Autodesk Fusion 360 part; units mm, degrees
(part 2 of 7)
  spline S300 degree 3 poles (-43.8986, 66.1485) (-43.8986, 66.1919) (-43.9124, 66.232) (-43.9361, 66.2647) knots 0 0 0 0 1 1 1 1
  spline S301 degree 3 poles (-43.9361, 66.2647) (-43.9588, 66.2897) (-43.9916, 66.3058) (-44.0281, 66.3058) knots 0 0 0 0 1 1 1 1
  line L172 (-44.0281, 66.3058) -> (-44.0291, 66.3058)
  spline S302 degree 3 poles (-44.0291, 66.3058) (-44.0304, 66.3058) (-44.0321, 66.3058) (-44.0335, 66.3058) knots 0 0 0 0 1 1 1 1
  spline S303 degree 3 poles (-44.0335, 66.3058) (-44.0697, 66.3058) (-44.1018, 66.2891) (-44.1235, 66.263) knots 0 0 0 0 1 1 1 1
  spline S304 degree 3 poles (-44.1235, 66.263) (-44.1441, 66.2339) (-44.1563, 66.1974) (-44.1563, 66.1582) knots 0 0 0 0 1 1 1 1
  spline S305 degree 3 poles (-44.1563, 66.1582) (-44.1563, 66.1516) (-44.1559, 66.1451) (-44.1553, 66.1389) knots 0 0 0 0 1 1 1 1
  line L173 (-44.1553, 66.1389) -> (-44.1573, 66.0745)
  spline S306 degree 3 poles (-44.1573, 66.0745) (-44.1654, 65.7573) (-44.1749, 65.398) (-44.5986, 65.398) knots 0 0 0 0 1 1 1 1
  spline S307 degree 3 poles (-44.5986, 65.398) (-44.8049, 65.398) (-45.0251, 65.5306) (-45.0251, 65.9016) knots 0 0 0 0 1 1 1 1
  line L174 (-45.0251, 65.9016) -> (-45.0251, 66.6018)
  line L175 (-45.0251, 66.6018) -> (-44.72, 66.6018)
  line L176 (-44.72, 66.6018) -> (-44.72, 65.9614)
  spline S308 degree 3 poles (-44.72, 65.9614) (-44.721, 65.9534) (-44.7214, 65.9444) (-44.7214, 65.935) knots 0 0 0 0 1 1 1 1
  spline S309 degree 3 poles (-44.7214, 65.935) (-44.7214, 65.8927) (-44.7109, 65.853) (-44.6923, 65.8184) knots 0 0 0 0 1 1 1 1
  line L177 (-44.6923, 65.8184) -> (-44.693, 65.8198)
  spline S310 degree 3 poles (-44.693, 65.8198) (-44.673, 65.7889) (-44.6389, 65.7685) (-44.6007, 65.7685) knots 0 0 0 0 1 1 1 1
  spline S311 degree 3 poles (-44.6007, 65.7685) (-44.5973, 65.7685) (-44.5942, 65.7685) (-44.5909, 65.7687) knots 0 0 0 0 1 1 1 1
  line L178 (-44.5909, 65.7687) -> (-44.5875, 65.7687)
  spline S312 degree 3 poles (-44.5875, 65.7687) (-44.5395, 65.7687) (-44.4989, 65.8006) (-44.4847, 65.8451) knots 0 0 0 0 1 1 1 1
  spline S313 degree 3 poles (-44.4847, 65.8451) (-44.4738, 65.8802) (-44.4674, 65.9197) (-44.4674, 65.9606) knots 0 0 0 0 1 1 1 1
  spline S314 degree 3 poles (-44.4674, 65.9606) (-44.4674, 65.9677) (-44.4677, 65.9748) (-44.4681, 65.9818) knots 0 0 0 0 1 1 1 1
  line L179 (-44.4681, 65.9818) -> (-44.4681, 65.9807)
  line L180 (-44.4681, 65.9807) -> (-44.4633, 66.1712)
  spline S315 degree 3 poles (-44.4633, 66.1712) (-44.465, 66.1872) (-44.4661, 66.206) (-44.4661, 66.2247) knots 0 0 0 0 1 1 1 1
  spline S316 degree 3 poles (-44.4661, 66.2247) (-44.4661, 66.3556) (-44.4218, 66.476) (-44.3474, 66.5708) knots 0 0 0 0 1 1 1 1
  line L181 (-44.3474, 66.5708) -> (-44.348, 66.5696)
  spline S317 degree 3 poles (-44.348, 66.5696) (-44.3399, 66.5801) (-44.3311, 66.5891) (-44.3213, 66.5971) knots 0 0 0 0 1 1 1 1
  line L182 (-44.3213, 66.5971) -> (-43.7758, 66.6017)
  spline S318 degree 3 poles (-43.7758, 66.6017) (-43.6615, 66.5006) (-43.5895, 66.3517) (-43.5895, 66.1855) knots 0 0 0 0 1 1 1 1
  spline S319 degree 3 poles (-43.5895, 66.1855) (-43.5895, 66.164) (-43.5908, 66.1428) (-43.5929, 66.1223) knots 0 0 0 0 1 1 1 1
  line L183 (-43.5929, 66.1223) -> (-43.5925, 66.1249)
  line L184 (-43.5925, 64.7542) -> (-43.5925, 64.0697)
  line L185 (-43.5925, 64.0697) -> (-43.9003, 64.0697)
  line L186 (-43.9003, 64.0697) -> (-43.9003, 64.7506)
  spline S320 degree 3 poles (-43.9003, 64.7506) (-43.8993, 64.7583) (-43.8986, 64.7673) (-43.8986, 64.7764) knots 0 0 0 0 1 1 1 1
  spline S321 degree 3 poles (-43.8986, 64.7764) (-43.8986, 64.8205) (-43.9124, 64.8614) (-43.9361, 64.8948) knots 0 0 0 0 1 1 1 1
  spline S322 degree 3 poles (-43.9361, 64.8948) (-43.9588, 64.9194) (-43.9919, 64.935) (-44.0281, 64.935) knots 0 0 0 0 1 1 1 1
  line L187 (-44.0281, 64.935) -> (-44.0291, 64.935)
  spline S323 degree 3 poles (-44.0291, 64.935) (-44.0298, 64.935) (-44.0308, 64.935) (-44.0315, 64.935) knots 0 0 0 0 1 1 1 1
  spline S324 degree 3 poles (-44.0315, 64.935) (-44.068, 64.935) (-44.1012, 64.9183) (-44.1235, 64.8922) knots 0 0 0 0 1 1 1 1
  spline S325 degree 3 poles (-44.1235, 64.8922) (-44.1441, 64.8627) (-44.1563, 64.8257) (-44.1563, 64.7857) knots 0 0 0 0 1 1 1 1
  spline S326 degree 3 poles (-44.1563, 64.7857) (-44.1563, 64.7791) (-44.1559, 64.7725) (-44.1553, 64.7662) knots 0 0 0 0 1 1 1 1
  line L188 (-44.1553, 64.7662) -> (-44.1573, 64.7024)
  spline S327 degree 3 poles (-44.1573, 64.7024) (-44.1654, 64.3862) (-44.1749, 64.0274) (-44.5986, 64.0274) knots 0 0 0 0 1 1 1 1
  spline S328 degree 3 poles (-44.5986, 64.0274) (-44.8049, 64.0274) (-45.0251, 64.1593) (-45.0251, 64.5296) knots 0 0 0 0 1 1 1 1
  line L189 (-45.0251, 64.5296) -> (-45.0251, 65.2335)
  line L190 (-45.0251, 65.2335) -> (-44.72, 65.2335)
  line L191 (-44.72, 65.2335) -> (-44.72, 64.5894)
  spline S329 degree 3 poles (-44.72, 64.5894) (-44.7211, 64.5814) (-44.7214, 64.5724) (-44.7214, 64.5633) knots 0 0 0 0 1 1 1 1
  spline S330 degree 3 poles (-44.7214, 64.5633) (-44.7214, 64.5213) (-44.7109, 64.4818) (-44.6923, 64.4474) knots 0 0 0 0 1 1 1 1
  line L192 (-44.6923, 64.4474) -> (-44.693, 64.4489)
  spline S331 degree 3 poles (-44.693, 64.4489) (-44.671, 64.4165) (-44.6352, 64.3956) (-44.5946, 64.3956) knots 0 0 0 0 1 1 1 1
  spline S332 degree 3 poles (-44.5946, 64.3956) (-44.5445, 64.3956) (-44.5016, 64.4273) (-44.4837, 64.4717) knots 0 0 0 0 1 1 1 1
  spline S333 degree 3 poles (-44.4837, 64.4717) (-44.4728, 64.5072) (-44.4664, 64.5467) (-44.4664, 64.5881) knots 0 0 0 0 1 1 1 1
  spline S334 degree 3 poles (-44.4664, 64.5881) (-44.4664, 64.5954) (-44.4667, 64.6029) (-44.4671, 64.6103) knots 0 0 0 0 1 1 1 1
  line L193 (-44.4671, 64.6103) -> (-44.4671, 64.6091)
  line L194 (-44.4671, 64.6091) -> (-44.4624, 64.7984)
  spline S335 degree 3 poles (-44.4624, 64.7984) (-44.4641, 64.8143) (-44.4647, 64.8327) (-44.4647, 64.8511) knots 0 0 0 0 1 1 1 1
  spline S336 degree 3 poles (-44.4647, 64.8511) (-44.4647, 64.9829) (-44.4204, 65.1044) (-44.346, 65.2003) knots 0 0 0 0 1 1 1 1
  line L195 (-44.346, 65.2003) -> (-44.347, 65.1991)
  spline S337 degree 3 poles (-44.347, 65.1991) (-44.276, 65.2652) (-44.1817, 65.3058) (-44.0778, 65.3058) knots 0 0 0 0 1 1 1 1
  spline S338 degree 3 poles (-44.0778, 65.3058) (-44.066, 65.3058) (-44.0538, 65.3049) (-44.0423, 65.304) knots 0 0 0 0 1 1 1 1
  line L196 (-44.0423, 65.304) -> (-44.044, 65.304)
  spline S339 degree 3 poles (-44.044, 65.304) (-43.7454, 65.3049) (-43.5932, 65.1193) (-43.5932, 64.7531) knots 0 0 0 0 1 1 1 1
  line L197 (-43.5932, 64.7531) -> (-43.5925, 64.7542)
  line L198 (-43.5925, 63.8593) -> (-43.5925, 62.6862)
  line L199 (-43.5925, 62.6862) -> (-45.0254, 62.6862)
  line L200 (-45.0254, 62.6862) -> (-45.0254, 63.8582)
  line L201 (-45.0254, 63.8582) -> (-44.7295, 63.8582)
  line L202 (-44.7295, 63.8582) -> (-44.7295, 63.0367)
  line L203 (-44.7295, 63.0367) -> (-44.4691, 63.0367)
  line L204 (-44.4691, 63.0367) -> (-44.4691, 63.8392)
  line L205 (-44.4691, 63.8392) -> (-44.1773, 63.8392)
  line L206 (-44.1773, 63.8392) -> (-44.1773, 63.0367)
  line L207 (-44.1773, 63.0367) -> (-43.8925, 63.0367)
  line L208 (-43.8925, 63.0367) -> (-43.8911, 63.8593)
  line L209 (-43.8911, 63.8593) -> (-43.5935, 63.8593)
  line L210 (-43.5935, 63.8593) -> (-43.5925, 63.8593)
  line L211 (-46.0566, 64.5431) -> (-46.0566, 63.8278)
  line L212 (-46.0566, 63.8278) -> (-46.3758, 63.691)
  line L213 (-46.3758, 63.691) -> (-46.3758, 62.9615)
  line L214 (-46.3758, 62.9615) -> (-46.0566, 62.8289)
  line L215 (-46.0566, 62.8289) -> (-46.0566, 62.4179)
  spline S340 degree 3 poles (-46.0566, 62.4179) (-46.0559, 62.4064) (-46.0556, 62.3929) (-46.0556, 62.3793) knots 0 0 0 0 1 1 1 1
  spline S341 degree 3 poles (-46.0556, 62.3793) (-46.0556, 62.2009) (-46.1154, 62.0368) (-46.2159, 61.907) knots 0 0 0 0 1 1 1 1
  line L216 (-46.2159, 61.907) -> (-46.2148, 61.9087)
  spline S342 degree 3 poles (-46.2148, 61.9087) (-46.3423, 61.7903) (-46.5118, 61.7181) (-46.6981, 61.7181) knots 0 0 0 0 1 1 1 1
  spline S343 degree 3 poles (-46.6981, 61.7181) (-46.7204, 61.7181) (-46.7428, 61.7192) (-46.7644, 61.7212) knots 0 0 0 0 1 1 1 1
  line L217 (-46.7644, 61.7212) -> (-46.7617, 61.721)
  spline S344 degree 3 poles (-46.7617, 61.721) (-46.7806, 61.7192) (-46.8026, 61.7181) (-46.8249, 61.7181) knots 0 0 0 0 1 1 1 1
  spline S345 degree 3 poles (-46.8249, 61.7181) (-47.0157, 61.7181) (-47.1895, 61.791) (-47.3221, 61.9111) knots 0 0 0 0 1 1 1 1
  spline S346 degree 3 poles (-47.3221, 61.9111) (-47.4269, 62.0343) (-47.4912, 62.1975) (-47.4912, 62.3763) knots 0 0 0 0 1 1 1 1
  spline S347 degree 3 poles (-47.4912, 62.3763) (-47.4912, 62.4002) (-47.4902, 62.4234) (-47.4878, 62.4467) knots 0 0 0 0 1 1 1 1
  line L218 (-47.4878, 62.4467) -> (-47.4881, 62.4438)
  line L219 (-47.4881, 62.4438) -> (-47.4881, 62.784)
  line L220 (-47.4881, 62.784) -> (-47.1827, 62.784)
  line L221 (-47.1827, 62.784) -> (-47.1827, 62.4508)
  spline S348 degree 3 poles (-47.1827, 62.4508) (-47.1844, 62.4384) (-47.1854, 62.4236) (-47.1854, 62.4088) knots 0 0 0 0 1 1 1 1
  spline S349 degree 3 poles (-47.1854, 62.4088) (-47.1854, 62.3203) (-47.1523, 62.2402) (-47.0979, 62.1801) knots 0 0 0 0 1 1 1 1
  spline S350 degree 3 poles (-47.0979, 62.1801) (-47.0187, 62.1165) (-46.9173, 62.0781) (-46.8074, 62.0781) knots 0 0 0 0 1 1 1 1
  spline S351 degree 3 poles (-46.8074, 62.0781) (-46.7955, 62.0781) (-46.7837, 62.0783) (-46.7722, 62.0792) knots 0 0 0 0 1 1 1 1
  line L222 (-46.7722, 62.0792) -> (-46.7739, 62.0792)
  spline S352 degree 3 poles (-46.7739, 62.0792) (-46.761, 62.0781) (-46.7458, 62.0772) (-46.7306, 62.0772) knots 0 0 0 0 1 1 1 1
  spline S353 degree 3 poles (-46.7306, 62.0772) (-46.6203, 62.0772) (-46.5185, 62.1144) (-46.4364, 62.1768) knots 0 0 0 0 1 1 1 1
  line L223 (-46.4364, 62.1768) -> (-46.4377, 62.1757)
  spline S354 degree 3 poles (-46.4377, 62.1757) (-46.391, 62.2344) (-46.3626, 62.3096) (-46.3626, 62.3922) knots 0 0 0 0 1 1 1 1
  spline S355 degree 3 poles (-46.3626, 62.3922) (-46.3626, 62.4023) (-46.363, 62.4121) (-46.364, 62.4217) knots 0 0 0 0 1 1 1 1
  line L224 (-46.364, 62.4217) -> (-46.364, 62.4203)
  line L225 (-46.364, 62.4203) -> (-46.364, 62.578)
  line L226 (-46.364, 62.578) -> (-47.4902, 63.0747)
  line L227 (-47.4902, 63.0747) -> (-47.4902, 63.6022)
  line L228 (-47.4902, 63.6022) -> (-46.1374, 64.1968)
  line L229 (-46.1374, 64.1968) -> (-47.4902, 64.1968)
  line L230 (-47.4902, 64.1968) -> (-47.4902, 64.7316)
  line L231 (-47.4902, 64.7316) -> (-46.4932, 65.3489)
  line L232 (-46.4932, 65.3489) -> (-47.4902, 65.3489)
  line L233 (-47.4902, 65.3489) -> (-47.4902, 65.7097)
  line L234 (-47.4902, 65.7097) -> (-46.059, 65.7097)
  line L235 (-46.059, 65.7097) -> (-46.059, 65.2088)
  line L236 (-46.059, 65.2088) -> (-47.1337, 64.5423)
  line L237 (-47.1337, 64.5423) -> (-46.059, 64.5423)
  line L238 (-46.059, 64.5423) -> (-46.0566, 64.5431)
  line L239 (-47.2463, 63.3286) -> (-46.6755, 63.0867)
  line L240 (-46.6755, 63.0867) -> (-46.6755, 63.5715)
  line L241 (-46.6755, 63.5715) -> (-47.2463, 63.3286)
  line L242 (-46.0573, 59.9275) -> (-46.0573, 59.5762)
  line L243 (-46.0573, 59.5762) -> (-47.4892, 59.5762)
  line L244 (-47.4892, 59.5762) -> (-47.4892, 60.3842)
  spline S356 degree 3 poles (-47.4892, 60.3842) (-47.4919, 60.4092) (-47.4932, 60.4384) (-47.4932, 60.4679) knots 0 0 0 0 1 1 1 1
  spline S357 degree 3 poles (-47.4932, 60.4679) (-47.4932, 60.5917) (-47.4665, 60.7095) (-47.4185, 60.815) knots 0 0 0 0 1 1 1 1
  line L245 (-47.4185, 60.815) -> (-47.4205, 60.8097)
  spline S358 degree 3 poles (-47.4205, 60.8097) (-47.362, 60.917) (-47.2521, 60.9882) (-47.1259, 60.9882) knots 0 0 0 0 1 1 1 1
  spline S359 degree 3 poles (-47.1259, 60.9882) (-47.1178, 60.9882) (-47.11, 60.9879) (-47.1023, 60.9873) knots 0 0 0 0 1 1 1 1
  line L246 (-47.1023, 60.9873) -> (-47.1033, 60.9873)
  line L247 (-47.1033, 60.9873) -> (-47.0928, 60.9873)
  spline S360 degree 3 poles (-47.0928, 60.9873) (-46.9281, 60.9873) (-46.7864, 60.8867) (-46.7228, 60.7423) knots 0 0 0 0 1 1 1 1
  line L248 (-46.7228, 60.7423) -> (-46.7218, 60.7394)
  spline S361 degree 3 poles (-46.7218, 60.7394) (-46.6961, 60.8092) (-46.6548, 60.8679) (-46.6021, 60.9126) knots 0 0 0 0 1 1 1 1
  line L249 (-46.6021, 60.9126) -> (-46.6014, 60.9134)
  spline S362 degree 3 poles (-46.6014, 60.9134) (-46.5405, 60.9515) (-46.4668, 60.9745) (-46.3877, 60.9745) knots 0 0 0 0 1 1 1 1
  spline S363 degree 3 poles (-46.3877, 60.9745) (-46.3704, 60.9745) (-46.3535, 60.9733) (-46.3366, 60.9713) knots 0 0 0 0 1 1 1 1
  line L250 (-46.3366, 60.9713) -> (-46.3386, 60.9716)
  line L251 (-46.3386, 60.9716) -> (-46.0576, 60.9716)
  line L252 (-46.0576, 60.9716) -> (-46.0576, 60.6173)
  line L253 (-46.0576, 60.6173) -> (-46.2382, 60.6158)
  line L254 (-46.2382, 60.6158) -> (-46.2652, 60.6158)
  spline S364 degree 3 poles (-46.2652, 60.6158) (-46.2805, 60.6179) (-46.298, 60.6194) (-46.3163, 60.6194) knots 0 0 0 0 1 1 1 1
  spline S365 degree 3 poles (-46.3163, 60.6194) (-46.3907, 60.6194) (-46.46, 60.5975) (-46.5185, 60.5594) knots 0 0 0 0 1 1 1 1
  line L255 (-46.5185, 60.5594) -> (-46.5169, 60.5603)
  spline S366 degree 3 poles (-46.5169, 60.5603) (-46.5574, 60.5037) (-46.5821, 60.4325) (-46.5821, 60.3555) knots 0 0 0 0 1 1 1 1
  spline S367 degree 3 poles (-46.5821, 60.3555) (-46.5821, 60.3374) (-46.5808, 60.3195) (-46.5781, 60.302) knots 0 0 0 0 1 1 1 1
  line L256 (-46.5781, 60.302) -> (-46.5784, 60.3043)
  line L257 (-46.5784, 60.3043) -> (-46.5784, 59.9277)
  line L258 (-46.5784, 59.9277) -> (-46.0573, 59.9275)
  line L259 (-47.1912, 59.9275) -> (-46.8733, 59.9275)
  line L260 (-46.8733, 59.9275) -> (-46.8733, 60.3536)
  spline S368 degree 3 poles (-46.8733, 60.3536) (-46.8723, 60.3638) (-46.8716, 60.3757) (-46.8716, 60.3873) knots 0 0 0 0 1 1 1 1
  spline S369 degree 3 poles (-46.8716, 60.3873) (-46.8716, 60.4384) (-46.8831, 60.4863) (-46.9038, 60.529) knots 0 0 0 0 1 1 1 1
  line L261 (-46.9038, 60.529) -> (-46.9031, 60.5272)
  spline S370 degree 3 poles (-46.9031, 60.5272) (-46.9295, 60.5713) (-46.9761, 60.6002) (-47.0292, 60.6002) knots 0 0 0 0 1 1 1 1
  spline S371 degree 3 poles (-47.0292, 60.6002) (-47.0323, 60.6002) (-47.0356, 60.6002) (-47.0387, 60.5996) knots 0 0 0 0 1 1 1 1
  spline S372 degree 3 poles (-47.0387, 60.5996) (-47.0414, 60.6002) (-47.0441, 60.6002) (-47.0472, 60.6002) knots 0 0 0 0 1 1 1 1
  spline S373 degree 3 poles (-47.0472, 60.6002) (-47.0982, 60.6002) (-47.1425, 60.5703) (-47.1645, 60.5265) knots 0 0 0 0 1 1 1 1
  spline S374 degree 3 poles (-47.1645, 60.5265) (-47.1824, 60.4842) (-47.1929, 60.4359) (-47.1929, 60.385) knots 0 0 0 0 1 1 1 1
  spline S375 degree 3 poles (-47.1929, 60.385) (-47.1929, 60.3759) (-47.1926, 60.3669) (-47.1919, 60.3582) knots 0 0 0 0 1 1 1 1
  line L262 (-47.1919, 60.3582) -> (-47.1919, 60.3593)
  line L263 (-47.1919, 60.3593) -> (-47.1912, 59.9275)
  line L264 (-46.0573, 56.208) -> (-46.0573, 55.4944)
  line L265 (-46.0573, 55.4944) -> (-46.3765, 55.3593)
  line L266 (-46.3765, 55.3593) -> (-46.3765, 54.6276)
  line L267 (-46.3765, 54.6276) -> (-46.0573, 54.4916)
  line L268 (-46.0573, 54.4916) -> (-46.0573, 54.1098)
  line L269 (-46.0573, 54.1098) -> (-47.4892, 54.7391)
  line L270 (-47.4892, 54.7391) -> (-47.4892, 55.2608)
  line L271 (-47.4892, 55.2608) -> (-46.134, 55.8581)
  line L272 (-46.134, 55.8581) -> (-47.4892, 55.8581)
  line L273 (-47.4892, 55.8581) -> (-47.4892, 56.4312)
  line L274 (-47.4892, 56.4312) -> (-46.5182, 56.8907)
  line L275 (-46.5182, 56.8907) -> (-47.4892, 57.3131)
  line L276 (-47.4892, 57.3131) -> (-47.4892, 57.898)
  line L277 (-47.4892, 57.898) -> (-46.0579, 57.898)
  line L278 (-46.0579, 57.898) -> (-46.0579, 57.537)
  line L279 (-46.0579, 57.537) -> (-47.178, 57.5364)
  line L280 (-47.178, 57.5364) -> (-46.0576, 57.0272)
  line L281 (-46.0576, 57.0272) -> (-46.0576, 56.719)
  line L282 (-46.0576, 56.719) -> (-47.1797, 56.2084)
  line L283 (-47.1797, 56.2084) -> (-46.0573, 56.208)
  line L284 (-47.2463, 54.9918) -> (-46.6755, 54.7526)
  line L285 (-46.6755, 54.7526) -> (-46.6755, 55.2322)
  line L286 (-46.6755, 55.2322) -> (-47.2463, 54.9918)
  line L287 (-46.0576, 61.5477) -> (-46.0576, 61.1895)
  line L288 (-46.0576, 61.1895) -> (-47.4892, 61.1895)
  line L289 (-47.4892, 61.1895) -> (-47.4892, 61.548)
  line L290 (-47.4892, 61.548) -> (-46.0576, 61.5477)
  line L291 (-46.0576, 59.3312) -> (-46.0576, 58.16)
  line L292 (-46.0576, 58.16) -> (-47.4892, 58.16)
  line L293 (-47.4892, 58.16) -> (-47.4892, 59.3332)
  line L294 (-47.4892, 59.3332) -> (-47.1916, 59.3332)
  line L295 (-47.1916, 59.3332) -> (-47.1916, 58.5114)
  line L296 (-47.1916, 58.5114) -> (-46.9335, 58.5114)
  line L297 (-46.9335, 58.5114) -> (-46.9335, 59.3135)
  line L298 (-46.9335, 59.3135) -> (-46.6396, 59.3135)
  line L299 (-46.6396, 59.3135) -> (-46.6396, 58.5106)
  line L300 (-46.6396, 58.5106) -> (-46.3535, 58.5106)
  line L301 (-46.3535, 58.5106) -> (-46.3535, 59.3326)
  line L302 (-46.3535, 59.3326) -> (-46.0579, 59.3326)
  line L303 (-46.0579, 59.3326) -> (-46.0576, 59.3312)
  ellipse E0 centre (-45.5414, 48.1762) end of major axis (-45.5414, 50.128) minor radius 1.9518
  spline S376 degree 3 poles (-45.5413, 52.5482) (-44.4633, 52.5482) (-43.5894, 51.6744) (-43.5894, 50.5965) knots 0 0 0 0 1 1 1 1
  spline S377 degree 3 poles (-43.5894, 50.5965) (-43.5894, 49.5184) (-44.4633, 48.6446) (-45.5413, 48.6446) knots 0 0 0 0 1 1 1 1
  spline S378 degree 3 poles (-45.5413, 48.6446) (-46.6193, 48.6446) (-47.4931, 49.5184) (-47.4931, 50.5965) knots 0 0 0 0 1 1 1 1
  spline S379 degree 3 poles (-47.4931, 50.5965) (-47.4931, 51.6744) (-46.6193, 52.5482) (-45.5413, 52.5482) knots 0 0 0 0 1 1 1 1
  spline S380 degree 3 poles (-47.0729, 49.3863) (-46.7154, 48.9344) (-46.1622, 48.6446) (-45.5413, 48.6446) knots 0 0 0 0 1 1 1 1
  spline S381 degree 3 poles (-45.5413, 48.6446) (-44.9205, 48.6446) (-44.3673, 48.9344) (-44.0098, 49.3863) knots 0 0 0 0 1 1 1 1
  spline S382 degree 3 poles (-44.0098, 49.3863) (-44.3673, 49.8381) (-44.9205, 50.128) (-45.5414, 50.128) knots 0 0 0 0 1 1 1 1
  spline S383 degree 3 poles (-45.5414, 50.128) (-46.1622, 50.128) (-46.7154, 49.8381) (-47.0729, 49.3863) knots 0 0 0 0 1 1 1 1
  spline S384 degree 3 poles (-46.3077, 38.5284) (-46.3077, 38.1545) (-46.5644, 37.8257) (-47.006, 37.8257) knots 0 0 0 0 1 1 1 1
  spline S385 degree 3 poles (-47.006, 37.8257) (-47.4464, 37.8257) (-47.7032, 38.1555) (-47.7032, 38.5284) knots 0 0 0 0 1 1 1 1
  spline S386 degree 3 poles (-47.7032, 38.5284) (-47.7032, 38.8981) (-47.4454, 39.227) (-47.006, 39.227) knots 0 0 0 0 1 1 1 1
  spline S387 degree 3 poles (-47.006, 39.227) (-46.5644, 39.2279) (-46.3077, 38.8981) (-46.3077, 38.5284) knots 0 0 0 0 1 1 1 1
  spline S388 degree 3 poles (-47.5409, 38.5285) (-47.5409, 38.249) (-47.3272, 38.0266) (-47.0059, 38.0266) knots 0 0 0 0 1 1 1 1
  spline S389 degree 3 poles (-47.0059, 38.0266) (-46.6847, 38.0266) (-46.4688, 38.249) (-46.4688, 38.5285) knots 0 0 0 0 1 1 1 1
  spline S390 degree 3 poles (-46.4688, 38.5285) (-46.4688, 38.7971) (-46.6847, 39.026) (-47.0059, 39.026) knots 0 0 0 0 1 1 1 1
  spline S391 degree 3 poles (-47.0059, 39.026) (-47.3272, 39.026) (-47.5409, 38.7971) (-47.5409, 38.5285) knots 0 0 0 0 1 1 1 1
  spline S392 degree 3 poles (-45.0228, 38.5327) (-46.1175, 37.4503) (-47.0023, 36.1744) (-47.6323, 34.7695) knots 0 0 0 0 1 1 1 1
  spline S393 degree 3 poles (-47.6323, 34.7695) (-48.2605, 33.3622) (-48.5856, 31.8384) (-48.5863, 30.2971) knots 0 0 0 0 1 1 1 1
  spline S394 degree 3 poles (-48.5863, 30.2971) (-48.5854, 28.5466) (-48.1674, 26.8215) (-47.3669, 25.2648) knots 0 0 0 0 1 1 1 1
  spline S395 degree 3 poles (-47.3669, 25.2648) (-46.5902, 23.7378) (-45.4837, 22.3687) (-44.0753, 21.1974) knots 0 0 0 0 1 1 1 1
  spline S396 degree 3 poles (-44.0753, 21.1974) (-41.2068, 18.8097) (-37.4027, 17.4944) (-33.3623, 17.4944) knots 0 0 0 0 1 1 1 1
  spline S397 degree 3 poles (-33.3623, 17.4944) (-28.8523, 17.4944) (-24.6024, 19.1589) (-21.7018, 22.0614) knots 0 0 0 0 1 1 1 1
  spline S398 degree 3 poles (-21.7018, 22.0614) (-20.6065, 23.1441) (-19.7215, 24.4204) (-19.0911, 25.8257) knots 0 0 0 0 1 1 1 1
  spline S399 degree 3 poles (-19.0911, 25.8257) (-18.4623, 27.2329) (-18.1373, 28.7569) (-18.1373, 30.2982) knots 0 0 0 0 1 1 1 1
  spline S400 degree 3 poles (-18.1373, 30.2982) (-18.1373, 31.8395) (-18.4623, 33.3636) (-19.0911, 34.7706) knots 0 0 0 0 1 1 1 1
  spline S401 degree 3 poles (-19.0911, 34.7706) (-19.6971, 36.1429) (-20.5769, 37.4088) (-21.7018, 38.5338) knots 0 0 0 0 1 1 1 1
  spline S402 degree 3 poles (-21.7018, 38.5338) (-24.6024, 41.4363) (-28.8523, 43.1009) (-33.3623, 43.1009) knots 0 0 0 0 1 1 1 1
  spline S403 degree 3 poles (-33.3623, 43.1009) (-37.8711, 43.0998) (-42.1211, 41.4352) (-45.0228, 38.5327) knots 0 0 0 0 1 1 1 1
  spline S404 degree 3 poles (-18.4058, 30.2971) (-18.4064, 31.8009) (-18.7229, 33.2877) (-19.335, 34.661) knots 0 0 0 0 1 1 1 1
  spline S405 degree 3 poles (-19.335, 34.661) (-19.952, 36.0356) (-20.8183, 37.2838) (-21.8898, 38.3427) knots 0 0 0 0 1 1 1 1
  spline S406 degree 3 poles (-21.8898, 38.3427) (-24.741, 41.1946) (-28.9232, 42.8323) (-33.3623, 42.8323) knots 0 0 0 0 1 1 1 1
  spline S407 degree 3 poles (-33.3623, 42.8323) (-37.8002, 42.8323) (-41.9804, 41.1957) (-44.8327, 38.3427) knots 0 0 0 0 1 1 1 1
  spline S408 degree 3 poles (-44.8327, 38.3427) (-45.9051, 37.2846) (-46.7714, 36.0361) (-47.3874, 34.661) knots 0 0 0 0 1 1 1 1
  spline S409 degree 3 poles (-47.3874, 34.661) (-48.0422, 33.1946) (-48.3589, 31.5995) (-48.3139, 29.994) knots 0 0 0 0 1 1 1 1
  spline S410 degree 3 poles (-48.3139, 29.994) (-48.2689, 28.3885) (-47.8634, 26.8137) (-47.1274, 25.3862) knots 0 0 0 0 1 1 1 1
  spline S411 degree 3 poles (-47.1274, 25.3862) (-46.3678, 23.8936) (-45.2839, 22.5536) (-43.9023, 21.4027) knots 0 0 0 0 1 1 1 1
  spline S412 degree 3 poles (-43.9023, 21.4027) (-41.0833, 19.0558) (-37.3394, 17.7631) (-33.3623, 17.7631) knots 0 0 0 0 1 1 1 1
  spline S413 degree 3 poles (-33.3623, 17.7631) (-28.9232, 17.7631) (-24.742, 19.3986) (-21.8898, 22.2517) knots 0 0 0 0 1 1 1 1
  spline S414 degree 3 poles (-21.8898, 22.2517) (-20.8184, 23.3107) (-19.9523, 24.5589) (-19.335, 25.9332) knots 0 0 0 0 1 1 1 1
  spline S415 degree 3 poles (-19.335, 25.9332) (-18.7229, 27.3066) (-18.4064, 28.7934) (-18.4058, 30.2971) knots 0 0 0 0 1 1 1 1
  spline S416 degree 3 poles (-44.5598, 38.0686) (-45.5975, 37.0437) (-46.4367, 35.8356) (-47.035, 34.5053) knots 0 0 0 0 1 1 1 1
  spline S417 degree 3 poles (-47.035, 34.5053) (-47.6658, 33.0909) (-47.9708, 31.5528) (-47.9272, 30.0047) knots 0 0 0 0 1 1 1 1
  spline S418 degree 3 poles (-47.9272, 30.0047) (-47.8837, 28.4566) (-47.4929, 26.9381) (-46.7836, 25.5614) knots 0 0 0 0 1 1 1 1
  spline S419 degree 3 poles (-46.7836, 25.5614) (-46.0488, 24.1139) (-44.9959, 22.8158) (-43.6563, 21.7004) knots 0 0 0 0 1 1 1 1
  spline S420 degree 3 poles (-43.6563, 21.7004) (-40.9061, 19.4104) (-37.2491, 18.1499) (-33.3623, 18.1499) knots 0 0 0 0 1 1 1 1
  spline S421 degree 3 poles (-33.3623, 18.1499) (-29.0242, 18.1499) (-24.944, 19.7446) (-22.1647, 22.5246) knots 0 0 0 0 1 1 1 1
  spline S422 degree 3 poles (-22.1647, 22.5246) (-21.1257, 23.5497) (-20.2858, 24.7587) (-19.6874, 26.0901) knots 0 0 0 0 1 1 1 1
  spline S423 degree 3 poles (-19.6874, 26.0901) (-19.0967, 27.414) (-18.791, 28.8474) (-18.7904, 30.2972) knots 0 0 0 0 1 1 1 1
  spline S424 degree 3 poles (-18.7904, 30.2972) (-18.791, 31.7473) (-19.0966, 33.181) (-19.6874, 34.5053) knots 0 0 0 0 1 1 1 1
  spline S425 degree 3 poles (-19.6874, 34.5053) (-20.2861, 35.8359) (-21.126, 37.044) (-22.1647, 38.0686) knots 0 0 0 0 1 1 1 1
  spline S426 degree 3 poles (-22.1647, 38.0686) (-24.944, 40.8497) (-29.0242, 42.4444) (-33.3623, 42.4444) knots 0 0 0 0 1 1 1 1
  spline S427 degree 3 poles (-33.3623, 42.4444) (-37.6993, 42.4455) (-41.7805, 40.8497) (-44.5598, 38.0686) knots 0 0 0 0 1 1 1 1
  spline S428 degree 3 poles (-39.2258, 34.8556) (-39.2258, 33.5058) (-38.2192, 30.2176) (-38.1784, 30.0779) knots 0 0 0 0 1 1 1 1
  spline S429 degree 3 poles (-38.1784, 30.0779) (-38.1742, 30.0631) (-38.1673, 30.0492) (-38.158, 30.037) knots 0 0 0 0 1 1 1 1
  line L304 (-38.158, 30.037) -> (-38.1622, 30.0349)
  spline S430 degree 3 poles (-38.1622, 30.0349) (-38.8343, 29.8896) (-39.4862, 29.663) (-40.1035, 29.36) knots 0 0 0 0 1 1 1 1
  spline S431 degree 3 poles (-40.1035, 29.36) (-40.3807, 30.0188) (-41.7085, 33.3361) (-41.5377, 35.9645) knots 0 0 0 0 1 1 1 1
  spline S432 degree 3 poles (-41.5377, 35.9645) (-40.3947, 37.2809) (-39.0034, 37.5613) (-38.7725, 37.5613) knots 0 0 0 0 1 1 1 1
  spline S433 degree 3 poles (-38.7725, 37.5613) (-38.7187, 37.5613) (-38.6693, 37.5571) (-38.6242, 37.5505) knots 0 0 0 0 1 1 1 1
  spline S434 degree 3 poles (-38.6242, 37.5505) (-38.9207, 37.0788) (-39.2258, 36.1386) (-39.2258, 34.8556) knots 0 0 0 0 1 1 1 1
  spline S435 degree 3 poles (-41.9116, 24.8564) (-42.4025, 25.1799) (-42.7109, 25.384) (-43.2115, 25.9127) knots 0 0 0 0 1 1 1 1
  spline S436 degree 3 poles (-43.2115, 25.9127) (-44.5264, 27.3011) (-45.4117, 29.1172) (-45.8822, 31.3308) knots 0 0 0 0 1 1 1 1
  spline S437 degree 2 poles (-45.8822, 31.3308) (-45.8983, 31.4157) (-45.8188, 31.4179) knots 0 0 0 1 1 1
  line L305 (-45.8188, 31.4179) -> (-44.1279, 31.3523)
  spline S438 degree 3 poles (-44.1279, 31.3523) (-44.1279, 31.0418) (-44.1193, 30.7409) (-44.101, 30.4443) knots 0 0 0 0 1 1 1 1
  spline S439 degree 3 poles (-44.101, 30.4443) (-44.1676, 30.6721) (-44.3116, 30.886) (-44.3675, 31.1213) knots 0 0 0 0 1 1 1 1
  spline S440 degree 3 poles (-44.3675, 31.1213) (-44.2525, 30.6345) (-44.1934, 30.1423) (-44.0344, 29.6921) knots 0 0 0 0 1 1 1 1
  spline S441 degree 3 poles (-44.0344, 29.6921) (-43.9968, 29.3815) (-43.9485, 29.0806) (-43.8905, 28.7894) knots 0 0 0 0 1 1 1 1
  spline S442 degree 3 poles (-43.8905, 28.7894) (-44.1827, 29.4331) (-44.506, 30.1069) (-44.6962, 30.8441) knots 0 0 0 0 1 1 1 1
  spline S443 degree 3 poles (-44.6962, 30.8441) (-44.4373, 29.835) (-44.159, 28.8818) (-43.7111, 28.048) knots 0 0 0 0 1 1 1 1
  spline S444 degree 3 poles (-43.7111, 28.048) (-43.6206, 27.7257) (-43.5108, 27.4092) (-43.3823, 27.1002) knots 0 0 0 0 1 1 1 1
  spline S445 degree 3 poles (-43.3823, 27.1002) (-44.0656, 28.0802) (-44.6747, 29.1978) (-45.0389, 30.4841) knots 0 0 0 0 1 1 1 1
  spline S446 degree 3 poles (-45.0389, 30.4841) (-44.5898, 28.8969) (-43.8206, 27.2528) (-42.8935, 26.1234) knots 0 0 0 0 1 1 1 1
  spline S447 degree 3 poles (-42.8935, 26.1234) (-43.7905, 27.026) (-44.4448, 27.9297) (-44.9497, 29.1494) knots 0 0 0 0 1 1 1 1
  spline S448 degree 3 poles (-44.9497, 29.1494) (-44.2536, 27.4451) (-43.1728, 25.8966) (-41.9116, 24.8564) knots 0 0 0 0 1 1 1 1
  spline S449 degree 3 poles (-42.5658, 26.1761) (-42.6367, 26.1761) (-42.684, 26.1922) (-42.7066, 26.2223) knots 0 0 0 0 1 1 1 1
  spline S450 degree 3 poles (-42.7066, 26.2223) (-42.7409, 26.2695) (-42.7313, 26.3534) (-42.7238, 26.3888) knots 0 0 0 0 1 1 1 1
  spline S451 degree 3 poles (-42.7238, 26.3888) (-42.6754, 26.4888) (-42.2575, 27.3452) (-41.6752, 27.9588) knots 0 0 0 0 1 1 1 1
  spline S452 degree 3 poles (-41.6752, 27.9588) (-40.3388, 29.3665) (-38.1343, 29.8007) (-38.1128, 29.805) knots 0 0 0 0 1 1 1 1
  line L306 (-38.1128, 29.805) -> (-38.1021, 29.8071)
  spline S453 degree 3 poles (-38.1021, 29.8071) (-37.0954, 30.1015) (-36.5132, 30.1864) (-36.3187, 30.0672) knots 0 0 0 0 1 1 1 1
  spline S454 degree 3 poles (-36.3187, 30.0672) (-36.2467, 30.0231) (-36.2285, 29.9446) (-36.2049, 29.8093) knots 0 0 0 0 1 1 1 1
  line L307 (-36.2049, 29.8093) -> (-36.2016, 29.7974)
  spline S455 degree 3 poles (-36.2016, 29.7974) (-36.1565, 29.5449) (-36.0491, 29.2311) (-35.9363, 28.8991) knots 0 0 0 0 1 1 1 1
  spline S456 degree 3 poles (-35.9363, 28.8991) (-35.8783, 28.7282) (-35.8181, 28.553) (-35.7622, 28.3736) knots 0 0 0 0 1 1 1 1
  spline S457 degree 3 poles (-35.7622, 28.3736) (-35.6591, 28.0426) (-35.8084, 27.9663) (-36.0663, 27.8814) knots 0 0 0 0 1 1 1 1
  spline S458 degree 3 poles (-36.0663, 27.8814) (-36.1017, 27.8696) (-36.135, 27.8589) (-36.164, 27.847) knots 0 0 0 0 1 1 1 1
  spline S459 degree 3 poles (-36.164, 27.847) (-39.3064, 26.5758) (-42.0663, 26.1761) (-42.5658, 26.1761) knots 0 0 0 0 1 1 1 1
  line L308 (-38.3481, 37.4206) -> (-38.3298, 37.3991)
  spline S460 degree 3 poles (-38.3298, 37.3991) (-38.2192, 37.2401) (-38.2858, 36.9918) (-38.3073, 36.9284) knots 0 0 0 0 1 1 1 1
  spline S461 degree 3 poles (-38.3073, 36.9284) (-38.3942, 36.9448) (-38.4787, 36.9723) (-38.5587, 37.0101) knots 0 0 0 0 1 1 1 1
  spline S462 degree 3 poles (-38.5587, 37.0101) (-38.4899, 37.1767) (-38.419, 37.3132) (-38.3481, 37.4206) knots 0 0 0 0 1 1 1 1
  spline S463 degree 3 poles (-42.3907, 29.6395) (-42.2285, 29.0904) (-41.9653, 28.6702) (-41.9524, 28.6326) knots 0 0 0 0 1 1 1 1
  spline S464 degree 3 poles (-41.9524, 28.6326) (-41.9556, 28.6422) (-42.0587, 29.1108) (-42.221, 29.662) knots 0 0 0 0 1 1 1 1
  spline S465 degree 3 poles (-42.221, 29.662) (-42.3843, 30.2122) (-42.6453, 31.2277) (-42.699, 31.621) knots 0 0 0 0 1 1 1 1
  spline S466 degree 3 poles (-42.699, 31.621) (-42.6453, 31.2191) (-42.554, 30.1875) (-42.3907, 29.6395) knots 0 0 0 0 1 1 1 1
  spline S467 degree 3 poles (-42.1511, 29.8512) (-41.9879, 29.302) (-41.7246, 28.883) (-41.7117, 28.8443) knots 0 0 0 0 1 1 1 1
  spline S468 degree 3 poles (-41.7117, 28.8443) (-41.7139, 28.8529) (-41.8181, 29.3235) (-41.9803, 29.8727) knots 0 0 0 0 1 1 1 1
  spline S469 degree 3 poles (-41.9803, 29.8727) (-42.1447, 30.4229) (-42.4047, 31.4383) (-42.4595, 31.8338) knots 0 0 0 0 1 1 1 1
  spline S470 degree 3 poles (-42.4595, 31.8338) (-42.4036, 31.4308) (-42.3134, 30.3992) (-42.1511, 29.8512) knots 0 0 0 0 1 1 1 1
  spline S471 degree 3 poles (-41.8826, 29.9629) (-41.7193, 29.4149) (-41.4561, 28.9947) (-41.4432, 28.9571) knots 0 0 0 0 1 1 1 1
  spline S472 degree 3 poles (-41.4432, 28.9571) (-41.4453, 28.9668) (-41.5495, 29.4364) (-41.7117, 29.9866) knots 0 0 0 0 1 1 1 1
  spline S473 degree 3 poles (-41.7117, 29.9866) (-41.8761, 30.5367) (-42.1372, 31.5522) (-42.1909, 31.9466) knots 0 0 0 0 1 1 1 1
  spline S474 degree 3 poles (-42.1909, 31.9466) (-42.1361, 31.5436) (-42.0459, 30.512) (-41.8826, 29.9629) knots 0 0 0 0 1 1 1 1
  spline S475 degree 3 poles (-41.6129, 30.122) (-41.4496, 29.5728) (-41.1875, 29.1527) (-41.1746, 29.1151) knots 0 0 0 0 1 1 1 1
  spline S476 degree 3 poles (-41.1746, 29.1151) (-41.1767, 29.1247) (-41.2799, 29.5943) (-41.4432, 30.1445) knots 0 0 0 0 1 1 1 1
  spline S477 degree 3 poles (-41.4432, 30.1445) (-41.6075, 30.6958) (-41.8675, 31.7102) (-41.9223, 32.1067) knots 0 0 0 0 1 1 1 1
  spline S478 degree 3 poles (-41.9223, 32.1067) (-41.8664, 31.7038) (-41.7751, 30.67) (-41.6129, 30.122) knots 0 0 0 0 1 1 1 1
  spline S479 degree 3 poles (-41.4346, 30.4583) (-41.2713, 29.9103) (-41.0081, 29.4901) (-40.9952, 29.4525) knots 0 0 0 0 1 1 1 1
  spline S480 degree 3 poles (-40.9952, 29.4525) (-40.9973, 29.4611) (-41.1015, 29.9318) (-41.2638, 30.482) knots 0 0 0 0 1 1 1 1
  spline S481 degree 3 poles (-41.2638, 30.482) (-41.4477, 31.1268) (-41.5965, 31.7811) (-41.7096, 32.442) knots 0 0 0 0 1 1 1 1
  spline S482 degree 3 poles (-41.7096, 32.442) (-41.6548, 32.039) (-41.5968, 31.0074) (-41.4346, 30.4583) knots 0 0 0 0 1 1 1 1
  spline S483 degree 3 poles (-41.1477, 30.6926) (-40.9995, 30.2004) (-40.7599, 29.8232) (-40.7481, 29.7899) knots 0 0 0 0 1 1 1 1
  spline S484 degree 3 poles (-40.7481, 29.7899) (-40.7502, 29.7974) (-40.8448, 30.2198) (-40.9941, 30.7141) knots 0 0 0 0 1 1 1 1
  spline S485 degree 3 poles (-40.9941, 30.7141) (-41.1445, 31.2073) (-41.3411, 32.1186) (-41.3916, 32.471) knots 0 0 0 0 1 1 1 1
  spline S486 degree 3 poles (-41.3916, 32.471) (-41.34, 32.111) (-41.2971, 31.1858) (-41.1477, 30.6926) knots 0 0 0 0 1 1 1 1
  spline S487 degree 3 poles (-42.5594, 29.2311) (-42.4412, 28.8045) (-42.2478, 28.4789) (-42.2392, 28.4499) knots 0 0 0 0 1 1 1 1
  spline S488 degree 3 poles (-42.2392, 28.4499) (-42.2414, 28.4563) (-42.3155, 28.8217) (-42.4358, 29.2483) knots 0 0 0 0 1 1 1 1
  spline S489 degree 3 poles (-42.4358, 29.2483) (-42.5562, 29.676) (-42.7946, 30.4648) (-42.8344, 30.771) knots 0 0 0 0 1 1 1 1
  spline S490 degree 3 poles (-42.8344, 30.771) (-42.7936, 30.4583) (-42.6786, 29.6567) (-42.5594, 29.2311) knots 0 0 0 0 1 1 1 1
  spline S491 degree 3 poles (-38.9121, 25.5345) (-38.7778, 25.3303) (-38.6177, 25.1896) (-38.6091, 25.1756) knots 0 0 0 0 1 1 1 1
  spline S492 degree 3 poles (-38.6091, 25.1756) (-38.6113, 25.1788) (-38.6048, 25.3948) (-38.7391, 25.6001) knots 0 0 0 0 1 1 1 1
  spline S493 degree 3 poles (-38.7391, 25.6001) (-38.8745, 25.8032) (-39.2387, 26.1406) (-39.3096, 26.2943) knots 0 0 0 0 1 1 1 1
  spline S494 degree 3 poles (-39.3096, 26.2943) (-39.192, 26.0335) (-39.0593, 25.7798) (-38.9121, 25.5345) knots 0 0 0 0 1 1 1 1
  spline S495 degree 3 poles (-39.2688, 25.5463) (-39.1345, 25.3432) (-38.9755, 25.2025) (-38.9658, 25.1885) knots 0 0 0 0 1 1 1 1
  spline S496 degree 3 poles (-38.9658, 25.1885) (-38.968, 25.1917) (-38.9615, 25.4077) (-39.0958, 25.6119) knots 0 0 0 0 1 1 1 1
  spline S497 degree 3 poles (-39.0958, 25.6119) (-39.2312, 25.8161) (-39.5954, 26.1535) (-39.6663, 26.3072) knots 0 0 0 0 1 1 1 1
  spline S498 degree 3 poles (-39.6663, 26.3072) (-39.5487, 26.046) (-39.416, 25.792) (-39.2688, 25.5463) knots 0 0 0 0 1 1 1 1
  spline S499 degree 3 poles (-39.6351, 25.5023) (-39.5245, 25.3239) (-39.3934, 25.2003) (-39.3848, 25.1885) knots 0 0 0 0 1 1 1 1
  spline S500 degree 3 poles (-39.3848, 25.1885) (-39.387, 25.1906) (-39.3826, 25.3808) (-39.4933, 25.5592) knots 0 0 0 0 1 1 1 1
  spline S501 degree 3 poles (-39.4933, 25.5592) (-39.604, 25.7387) (-39.9037, 26.0342) (-39.9617, 26.1685) knots 0 0 0 0 1 1 1 1
  spline S502 degree 3 poles (-39.9617, 26.1685) (-39.8648, 25.9408) (-39.7558, 25.7184) (-39.6351, 25.5023) knots 0 0 0 0 1 1 1 1
  spline S503 degree 3 poles (-39.9488, 25.4281) (-39.8521, 25.268) (-39.7382, 25.1573) (-39.7318, 25.1477) knots 0 0 0 0 1 1 1 1
  spline S504 degree 3 poles (-39.7318, 25.1477) (-39.7329, 25.1498) (-39.7286, 25.3196) (-39.8253, 25.4797) knots 0 0 0 0 1 1 1 1
  spline S505 degree 3 poles (-39.8253, 25.4797) (-39.9209, 25.6409) (-40.183, 25.9063) (-40.2335, 26.0267) knots 0 0 0 0 1 1 1 1
  spline S506 degree 3 poles (-40.2335, 26.0267) (-40.1498, 25.822) (-40.0548, 25.6222) (-39.9488, 25.4281) knots 0 0 0 0 1 1 1 1
  spline S507 degree 3 poles (-40.3431, 25.4926) (-40.2668, 25.3572) (-40.1755, 25.2648) (-40.1701, 25.2551) knots 0 0 0 0 1 1 1 1
  spline S508 degree 3 poles (-40.1701, 25.2551) (-40.1712, 25.2573) (-40.168, 25.4002) (-40.2442, 25.5345) knots 0 0 0 0 1 1 1 1
  spline S509 degree 3 poles (-40.2442, 25.5345) (-40.3216, 25.6699) (-40.53, 25.8924) (-40.5698, 25.9934) knots 0 0 0 0 1 1 1 1
  spline S510 degree 3 poles (-40.5698, 25.9934) (-40.5289, 25.8902) (-40.4193, 25.6269) (-40.3431, 25.4926) knots 0 0 0 0 1 1 1 1
  spline S511 degree 3 poles (-40.7008, 25.4786) (-40.6245, 25.3443) (-40.5332, 25.2508) (-40.5279, 25.2422) knots 0 0 0 0 1 1 1 1
  spline S512 degree 3 poles (-40.5279, 25.2422) (-40.5289, 25.2444) (-40.5257, 25.3862) (-40.602, 25.5216) knots 0 0 0 0 1 1 1 1
  spline S513 degree 3 poles (-40.602, 25.5216) (-40.6772, 25.656) (-40.8878, 25.8795) (-40.9264, 25.9794) knots 0 0 0 0 1 1 1 1
  spline S514 degree 3 poles (-40.9264, 25.9794) (-40.8867, 25.8773) (-40.7771, 25.614) (-40.7008, 25.4786) knots 0 0 0 0 1 1 1 1
  spline S515 degree 3 poles (-41.2326, 25.7204) (-41.1843, 25.6269) (-41.1263, 25.5614) (-41.123, 25.5549) knots 0 0 0 0 1 1 1 1
  spline S516 degree 3 poles (-41.123, 25.5549) (-41.1241, 25.5571) (-41.122, 25.656) (-41.1692, 25.7494) knots 0 0 0 0 1 1 1 1
  spline S517 degree 3 poles (-41.1692, 25.7494) (-41.2186, 25.844) (-41.3519, 25.9987) (-41.3776, 26.0697) knots 0 0 0 0 1 1 1 1
  spline S518 degree 3 poles (-41.3776, 26.0697) (-41.3508, 25.9987) (-41.282, 25.8139) (-41.2326, 25.7204) knots 0 0 0 0 1 1 1 1
  spline S519 degree 3 poles (-43.2577, 27.9588) (-43.2222, 27.8589) (-43.1728, 27.7869) (-43.1706, 27.7804) knots 0 0 0 0 1 1 1 1
  spline S520 degree 3 poles (-43.1706, 27.7804) (-43.1706, 27.7815) (-43.1545, 27.8793) (-43.19, 27.9792) knots 0 0 0 0 1 1 1 1
  spline S521 degree 3 poles (-43.19, 27.9792) (-43.2265, 28.0792) (-43.3361, 28.2522) (-43.3522, 28.3252) knots 0 0 0 0 1 1 1 1
  spline S522 degree 3 poles (-43.3522, 28.3252) (-43.3361, 28.25) (-43.2921, 28.0587) (-43.2577, 27.9588) knots 0 0 0 0 1 1 1 1
  spline S523 degree 3 poles (-38.6371, 25.6914) (-38.5028, 25.4883) (-38.3438, 25.3465) (-38.3341, 25.3336) knots 0 0 0 0 1 1 1 1
  spline S524 degree 3 poles (-38.3341, 25.3336) (-38.3363, 25.3368) (-38.3298, 25.5528) (-38.4652, 25.757) knots 0 0 0 0 1 1 1 1
  spline S525 degree 3 poles (-38.4652, 25.757) (-38.5995, 25.9611) (-38.9637, 26.2986) (-39.0346, 26.4511) knots 0 0 0 0 1 1 1 1
  spline S526 degree 3 poles (-39.0346, 26.4511) (-38.9168, 26.1905) (-38.784, 25.9368) (-38.6371, 25.6914) knots 0 0 0 0 1 1 1 1
  spline S527 degree 3 poles (-38.4018, 25.8429) (-38.2675, 25.6388) (-38.1085, 25.498) (-38.0988, 25.484) knots 0 0 0 0 1 1 1 1
  spline S528 degree 3 poles (-38.0988, 25.484) (-38.101, 25.4872) (-38.0946, 25.7032) (-38.2299, 25.9074) knots 0 0 0 0 1 1 1 1
  spline S529 degree 3 poles (-38.2299, 25.9074) (-38.3642, 26.1116) (-38.7295, 26.449) (-38.7993, 26.6027) knots 0 0 0 0 1 1 1 1
  spline S530 degree 3 poles (-38.7993, 26.6027) (-38.6815, 26.342) (-38.5488, 26.0883) (-38.4018, 25.8429) knots 0 0 0 0 1 1 1 1
  spline S531 degree 3 poles (-38.087, 25.9171) (-37.9818, 25.757) (-37.855, 25.6463) (-37.8475, 25.6355) knots 0 0 0 0 1 1 1 1
  spline S532 degree 3 poles (-37.8475, 25.6355) (-37.8496, 25.6377) (-37.8442, 25.8075) (-37.9517, 25.9676) knots 0 0 0 0 1 1 1 1
  spline S533 degree 3 poles (-37.9517, 25.9676) (-38.0591, 26.1277) (-38.347, 26.392) (-38.4029, 26.5124) knots 0 0 0 0 1 1 1 1
  spline S534 degree 3 poles (-38.4029, 26.5124) (-38.3099, 26.3077) (-38.2044, 26.1089) (-38.087, 25.9171) knots 0 0 0 0 1 1 1 1
  spline S535 degree 3 poles (-37.6863, 25.9246) (-37.581, 25.7656) (-37.4543, 25.6549) (-37.4468, 25.6441) knots 0 0 0 0 1 1 1 1
  spline S536 degree 3 poles (-37.4468, 25.6441) (-37.4489, 25.6463) (-37.4435, 25.8161) (-37.5499, 25.9751) knots 0 0 0 0 1 1 1 1
  spline S537 degree 3 poles (-37.5499, 25.9751) (-37.6573, 26.1363) (-37.9463, 26.4006) (-38.0022, 26.521) knots 0 0 0 0 1 1 1 1
  spline S538 degree 3 poles (-38.0022, 26.521) (-37.9092, 26.3159) (-37.8037, 26.1167) (-37.6863, 25.9246) knots 0 0 0 0 1 1 1 1
  spline S539 degree 3 poles (-37.2802, 25.8644) (-37.1567, 25.7161) (-37.0181, 25.6194) (-37.0106, 25.6119) knots 0 0 0 0 1 1 1 1
  spline S540 degree 3 poles (-37.0106, 25.6119) (-37.0117, 25.614) (-37.0267, 25.7827) (-37.1492, 25.93) knots 0 0 0 0 1 1 1 1
  spline S541 degree 3 poles (-37.1492, 25.93) (-37.2738, 26.0772) (-37.5896, 26.3093) (-37.6584, 26.4221) knots 0 0 0 0 1 1 1 1
  spline S542 degree 3 poles (-37.6584, 26.4221) (-37.5442, 26.2285) (-37.4179, 26.0422) (-37.2802, 25.8644) knots 0 0 0 0 1 1 1 1
  spline S543 degree 3 poles (-42.7656, 28.9614) (-42.6679, 28.6089) (-42.511, 28.3392) (-42.5035, 28.3156) knots 0 0 0 0 1 1 1 1
  spline S544 degree 3 poles (-42.5035, 28.3156) (-42.5057, 28.3209) (-42.5669, 28.6229) (-42.6647, 28.9754) knots 0 0 0 0 1 1 1 1
  spline S545 degree 3 poles (-42.6647, 28.9754) (-42.7624, 29.3289) (-42.959, 29.9812) (-42.9913, 30.2337) knots 0 0 0 0 1 1 1 1
  spline S546 degree 3 poles (-42.9913, 30.2337) (-42.9579, 29.9758) (-42.8634, 29.3139) (-42.7656, 28.9614) knots 0 0 0 0 1 1 1 1
  spline S547 degree 3 poles (-42.9633, 28.8324) (-42.8881, 28.5971) (-42.7656, 28.4177) (-42.7592, 28.4026) knots 0 0 0 0 1 1 1 1
  spline S548 degree 3 poles (-42.7592, 28.4026) (-42.7614, 28.4048) (-42.8086, 28.6068) (-42.8849, 28.841) knots 0 0 0 0 1 1 1 1
  spline S549 degree 3 poles (-42.8849, 28.841) (-42.9612, 29.0764) (-43.1137, 29.5094) (-43.1395, 29.6792) knots 0 0 0 0 1 1 1 1
  spline S550 degree 3 poles (-43.1395, 29.6792) (-43.1126, 29.5073) (-43.0396, 29.0656) (-42.9633, 28.8324) knots 0 0 0 0 1 1 1 1
  spline S551 degree 3 poles (-40.9415, 30.9182) (-40.7932, 30.4261) (-40.5515, 30.0478) (-40.5418, 30.0145) knots 0 0 0 0 1 1 1 1
  spline S552 degree 3 poles (-40.5418, 30.0145) (-40.5429, 30.0188) (-40.5665, 30.1263) (-40.6084, 30.2918) knots 0 0 0 0 1 1 1 1
  spline S553 degree 3 poles (-40.6084, 30.2918) (-40.8429, 30.942) (-41.0469, 31.6029) (-41.2197, 32.2722) knots 0 0 0 0 1 1 1 1
  spline S554 degree 3 poles (-41.2197, 32.2722) (-41.151, 31.8402) (-41.0468, 31.2696) (-40.9415, 30.9182) knots 0 0 0 0 1 1 1 1
  spline S555 degree 3 poles (-43.6143, 32.5602) (-43.566, 32.4012) (-43.5273, 32.2959) (-43.5252, 32.2787) knots 0 0 0 0 1 1 1 1
  spline S556 degree 3 poles (-43.5252, 32.2787) (-43.5252, 32.283) (-43.5327, 32.4764) (-43.5531, 32.759) knots 0 0 0 0 1 1 1 1
  spline S557 degree 3 poles (-43.5531, 32.759) (-43.5751, 32.6932) (-43.5955, 32.627) (-43.6143, 32.5602) knots 0 0 0 0 1 1 1 1
  spline S558 degree 3 poles (-41.8664, 35.569) (-41.8417, 35.1972) (-41.7794, 34.9222) (-41.7794, 34.8932) knots 0 0 0 0 1 1 1 1
  spline S559 degree 3 poles (-41.7794, 34.8932) (-41.7794, 34.9018) (-41.7386, 35.2747) (-41.7139, 35.7583) knots 0 0 0 0 1 1 1 1
  line L309 (-41.7139, 35.7583) -> (-41.8664, 35.569)
  spline S560 degree 3 poles (-42.4552, 34.8072) (-42.4015, 34.4149) (-42.3101, 34.127) (-42.3069, 34.1001) knots 0 0 0 0 1 1 1 1
  spline S561 degree 3 poles (-42.3069, 34.1001) (-42.308, 34.1087) (-42.2962, 34.4988) (-42.3134, 35.0006) knots 0 0 0 0 1 1 1 1
  line L310 (-42.3134, 35.0006) -> (-42.4552, 34.8072)
  spline S562 degree 3 poles (-42.9945, 33.9852) (-42.9193, 33.6478) (-42.8269, 33.4103) (-42.8226, 33.3823) knots 0 0 0 0 1 1 1 1
  spline S563 degree 3 poles (-42.8226, 33.3823) (-42.8237, 33.3909) (-42.8355, 33.7325) (-42.8752, 34.1818) knots 0 0 0 0 1 1 1 1
  spline S564 degree 3 poles (-42.8752, 34.1818) (-42.916, 34.1173) (-42.9558, 34.0497) (-42.9945, 33.9852) knots 0 0 0 0 1 1 1 1
  spline S565 degree 3 poles (-42.7753, 34.3418) (-42.698, 33.9938) (-42.6023, 33.7455) (-42.5991, 33.7186) knots 0 0 0 0 1 1 1 1
  spline S566 degree 3 poles (-42.5991, 33.7186) (-42.6002, 33.725) (-42.6109, 34.0733) (-42.6528, 34.5267) knots 0 0 0 0 1 1 1 1
  spline S567 degree 3 poles (-42.6528, 34.5267) (-42.6947, 34.4655) (-42.7356, 34.4021) (-42.7753, 34.3418) knots 0 0 0 0 1 1 1 1
  spline S568 degree 3 poles (-43.2426, 33.521) (-43.1793, 33.2769) (-43.1159, 33.1136) (-43.1126, 33.0911) knots 0 0 0 0 1 1 1 1
  spline S569 degree 3 poles (-43.1126, 33.0911) (-43.1137, 33.0975) (-43.1234, 33.349) (-43.1502, 33.7037) knots 0 0 0 0 1 1 1 1
  spline S570 degree 3 poles (-43.1502, 33.7037) (-43.1828, 33.6435) (-43.2136, 33.5826) (-43.2426, 33.521) knots 0 0 0 0 1 1 1 1
  spline S571 degree 3 poles (-42.1329, 35.2359) (-42.1092, 34.8556) (-42.0437, 34.5773) (-42.0437, 34.5472) knots 0 0 0 0 1 1 1 1
  spline S572 degree 3 poles (-42.0437, 34.5472) (-42.0437, 34.5579) (-42.0018, 34.9394) (-41.9782, 35.4305) knots 0 0 0 0 1 1 1 1
  line L311 (-41.9782, 35.4305) -> (-42.1329, 35.2359)
  spline S573 degree 3 poles (-43.4414, 33.0695) (-43.378, 32.83) (-43.3168, 32.6731) (-43.3135, 32.6473) knots 0 0 0 0 1 1 1 1
  spline S574 degree 3 poles (-43.3135, 32.6473) (-43.3146, 32.6559) (-43.3232, 32.9159) (-43.3533, 33.2813) knots 0 0 0 0 1 1 1 1
  spline S575 degree 3 poles (-43.3533, 33.2813) (-43.3837, 33.2112) (-43.413, 33.1406) (-43.4414, 33.0695) knots 0 0 0 0 1 1 1 1
  spline S576 degree 2 poles (-30.3961, 31.3105) (-30.5197, 31.4577) (-30.5304, 31.534) knots 0 0 0 1 1 1
  spline S577 degree 3 poles (-30.5304, 31.534) (-30.5432, 31.6135) (-30.3961, 31.4996) (-30.3961, 31.3105) knots 0 0 0 0 1 1 1 1
  spline S578 degree 3 poles (-35.5925, 36.9779) (-35.7719, 36.8772) (-35.9551, 36.7834) (-36.1415, 36.6964) knots 0 0 0 0 1 1 1 1
  spline S579 degree 3 poles (-36.1415, 36.6964) (-36.2106, 36.6669) (-36.2801, 36.6383) (-36.3499, 36.6104) knots 0 0 0 0 1 1 1 1
  line L312 (-36.3499, 36.6104) -> (-36.3499, 36.6082)
  spline S580 degree 3 poles (-36.3499, 36.6082) (-36.5905, 36.4911) (-36.8978, 36.302) (-37.0944, 36.317) knots 0 0 0 0 1 1 1 1
  spline S581 degree 3 poles (-37.0944, 36.317) (-37.2899, 36.3341) (-37.3629, 36.3804) (-37.4081, 36.2729) knots 0 0 0 0 1 1 1 1
  spline S582 degree 3 poles (-37.4081, 36.2729) (-37.4521, 36.1677) (-37.5305, 36.0946) (-37.5026, 36.0656) knots 0 0 0 0 1 1 1 1
  spline S583 degree 3 poles (-37.5026, 36.0656) (-37.4747, 36.0409) (-37.4295, 35.9001) (-37.4747, 35.8699) knots 0 0 0 0 1 1 1 1
  spline S584 degree 3 poles (-37.4747, 35.8699) (-37.5198, 35.8431) (-37.5585, 35.7647) (-37.5424, 35.7206) knots 0 0 0 0 1 1 1 1
  spline S585 degree 2 poles (-37.5424, 35.7206) (-37.4349, 35.8087) (-37.3737, 35.6852) knots 0 0 0 1 1 1
  spline S586 degree 3 poles (-37.3737, 35.6852) (-37.3125, 35.5615) (-37.3339, 35.5239) (-37.2953, 35.5175) knots 0 0 0 0 1 1 1 1
  spline S587 degree 3 poles (-37.2953, 35.5175) (-37.2566, 35.5111) (-37.2673, 35.3434) (-37.2168, 35.3682) knots 0 0 0 0 1 1 1 1
  spline S588 degree 3 poles (-37.2168, 35.3682) (-37.1663, 35.3896) (-37.0772, 35.4433) (-37.0718, 35.4015) knots 0 0 0 0 1 1 1 1
  spline S589 degree 3 poles (-37.0718, 35.4015) (-37.0229, 35.2527) (-36.9588, 35.1095) (-36.8806, 34.9738) knots 0 0 0 0 1 1 1 1
  spline S590 degree 3 poles (-36.8806, 34.9738) (-36.7968, 34.8309) (-36.8763, 35.0704) (-36.9257, 35.1983) knots 0 0 0 0 1 1 1 1
  spline S591 degree 3 poles (-36.9257, 35.1983) (-36.9762, 35.3262) (-36.7807, 35.2381) (-36.7463, 35.1501) knots 0 0 0 0 1 1 1 1
  spline S592 degree 3 poles (-36.7463, 35.1501) (-36.713, 35.0576) (-36.5626, 34.7717) (-36.496, 34.6062) knots 0 0 0 0 1 1 1 1
  spline S593 degree 2 poles (-36.496, 34.6062) (-36.6926, 34.6213) (-36.6808, 34.5708) knots 0 0 0 1 1 1
  spline S594 degree 3 poles (-36.6808, 34.5708) (-36.67, 34.5203) (-36.7817, 34.5708) (-36.815, 34.6062) knots 0 0 0 0 1 1 1 1
  spline S595 degree 3 poles (-36.815, 34.6062) (-36.8483, 34.6374) (-36.9214, 34.6374) (-36.8988, 34.5052) knots 0 0 0 0 1 1 1 1
  spline S596 degree 3 poles (-36.8988, 34.5052) (-36.8763, 34.3709) (-36.8322, 34.3977) (-36.8322, 34.2033) knots 0 0 0 0 1 1 1 1
  spline S597 degree 3 poles (-36.8322, 34.2033) (-36.8335, 33.9401) (-36.9152, 33.6837) (-37.0664, 33.4682) knots 0 0 0 0 1 1 1 1
  spline S598 degree 2 poles (-37.0664, 33.4682) (-37.0611, 33.4371) (-37.0611, 33.2899) knots 0 0 0 1 1 1
  spline S599 degree 3 poles (-37.0611, 33.2899) (-37.0611, 33.1426) (-36.8602, 33.0781) (-36.8602, 33.2436) knots 0 0 0 0 1 1 1 1
  spline S600 degree 2 poles (-36.8602, 33.2436) (-36.7925, 33.3339) (-36.7377, 33.2223) knots 0 0 0 1 1 1
  spline S601 degree 2 poles (-36.7377, 33.2223) (-36.6808, 33.1094) (-36.8269, 33.1094) knots 0 0 0 1 1 1
  spline S602 degree 2 poles (-36.8269, 33.1094) (-36.8269, 32.874) (-36.7033, 32.5968) knots 0 0 0 1 1 1
  spline S603 degree 2 poles (-36.7033, 32.5968) (-36.815, 32.7312) (-36.9386, 32.8192) knots 0 0 0 1 1 1
  spline S604 degree 2 poles (-36.9386, 32.8192) (-36.9268, 32.5968) (-36.8269, 32.4055) knots 0 0 0 1 1 1
  spline S605 degree 2 poles (-36.8269, 32.4055) (-37.3082, 32.974) (-37.5531, 34.0281) knots 0 0 0 1 1 1
  spline S606 degree 2 poles (-37.5531, 34.0281) (-37.6423, 33.839) (-37.5198, 33.3339) knots 0 0 0 1 1 1
  spline S607 degree 2 poles (-37.5198, 33.3339) (-37.8109, 33.7143) (-37.7658, 34.3312) knots 0 0 0 1 1 1
  spline S608 degree 2 poles (-37.7658, 34.3312) (-38.0118, 34.0055) (-38.1569, 33.983) knots 0 0 0 1 1 1
  line L313 (-38.1569, 33.983) -> (-38.1569, 33.5467)
  spline S609 degree 2 poles (-38.1569, 33.5467) (-38.2804, 33.5929) (-38.202, 33.2232) knots 0 0 0 1 1 1
  spline S610 degree 2 poles (-38.202, 33.2232) (-38.1236, 32.8536) (-38.101, 32.6526) knots 0 0 0 1 1 1
  spline S611 degree 2 poles (-38.101, 32.6526) (-38.1461, 33.3469) (-38.0118, 32.9654) knots 0 0 0 1 1 1
  spline S612 degree 3 poles (-38.0118, 32.9654) (-37.8775, 32.5849) (-37.4854, 31.4104) (-37.0492, 30.5927) knots 0 0 0 0 1 1 1 1
  spline S613 degree 2 poles (-37.0492, 30.5927) (-37.1728, 30.9741) (-37.1728, 31.1976) knots 0 0 0 1 1 1
  spline S614 degree 2 poles (-37.1728, 31.1976) (-36.8806, 30.7495) (-36.7366, 30.5486) knots 0 0 0 1 1 1
  line L314 (-36.7366, 30.5486) -> (-36.7581, 30.9064)
  spline S615 degree 2 poles (-36.7581, 30.9064) (-36.3219, 30.0887) (-36.4004, 30.6937) knots 0 0 0 1 1 1
  spline S616 degree 2 poles (-36.4004, 30.6937) (-35.9191, 29.8995) (-36.0534, 30.5593) knots 0 0 0 1 1 1
  spline S617 degree 2 poles (-36.0534, 30.5593) (-35.5495, 29.7426) (-35.8063, 30.6485) knots 0 0 0 1 1 1
  spline S618 degree 2 poles (-35.8063, 30.6485) (-35.1467, 29.4503) (-35.5377, 30.8162) knots 0 0 0 1 1 1
  spline S619 degree 2 poles (-35.5377, 30.8162) (-34.8899, 29.4396) (-35.2143, 30.8495) knots 0 0 0 1 1 1
  spline S620 degree 2 poles (-35.2143, 30.8495) (-34.5085, 29.5965) (-34.8329, 30.7485) knots 0 0 0 1 1 1
  spline S621 degree 2 poles (-34.8329, 30.7485) (-34.6213, 30.2896) (-34.14, 29.8189) knots 0 0 0 1 1 1
  spline S622 degree 2 poles (-34.14, 29.8189) (-34.7438, 31.0182) (-34.7664, 31.577) knots 0 0 0 1 1 1
  spline S623 degree 2 poles (-34.7664, 31.577) (-34.3968, 30.4906) (-33.692, 29.8093) knots 0 0 0 1 1 1
  spline S624 degree 2 poles (-33.692, 29.8093) (-34.2399, 30.6367) (-34.4419, 31.621) knots 0 0 0 1 1 1
  spline S625 degree 2 poles (-34.4419, 31.621) (-33.591, 29.7974) (-32.6962, 29.2376) knots 0 0 0 1 1 1
  line L315 (-32.6962, 29.2376) -> (-32.6962, 29.272)
  spline S626 degree 2 poles (-32.6962, 29.272) (-34.0831, 30.5916) (-34.2066, 32.0573) knots 0 0 0 1 1 1
  spline S627 degree 2 poles (-34.2066, 32.0573) (-33.6125, 30.0779) (-32.3491, 29.3042) knots 0 0 0 1 1 1